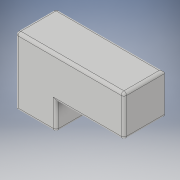
# Autodesk Inventor part: elbow
Saved by Autodesk Inventor 2019 (Build 230136000, 136)
## iProperties
Created: 2020-02-11
Part Number: elbow
Material: Generic
Document SubType Name: Modeling
Designer: Vinayak
Density: 1 g/cm^3
Appearance: Default
Author: Vinayak
Autodesk Inventor part; units mm, degrees
ref_plane "YZ Plane" through (0, 0, 0) normal (1, 0, 0) x (0, 1, 0)
ref_plane "XZ Plane" through (0, 0, 0) normal (0, 1, 0) x (-1, 0, 0)
ref_plane "XY Plane" through (0, 0, 0) normal (0, 0, 1) x (1, 0, 0)
sketch "Sketch1" plane through (0, 0, 0) normal (0, 0, 1) x (1, 0, 0)
  line L0 (0, 0) -> (-50, 0)
  line L1 (-50, 0) -> (-50, 30)
  line L2 (-50, 30) -> (0, 30)
  line L3 (0, 30) -> (0, 0)
  line L4 (-50, 30) -> (-80, 30)
  line L5 (-80, 30) -> (-80, -20)
  line L6 (-80, -20) -> (-50, -20)
  line L7 (-50, -20) -> (-50, 30)
  line L8 (-80, 0) -> (-50, 0)
  dimension "d0" = 50
  dimension "d1" = 30
  dimension "d2" = 30
  dimension "d3" = 50
  constraints: 18 end point, 4 parallel, 3 perpendicular, 2 horizontal, 1 point on line
  measures "d0" distance of L1.end L2.end
  measures "d1" distance of L0.end L1.end
  measures "d2" distance of L6.end L5.end
  measures "d3" distance of L5.end L4.end
extrude "Extrusion1" add sketch "Sketch1" along normal blind 30
fillet "Fillet1" radius 2 12 edges at (-40, 30, 30) (0, 15, 30) (-25, 0, 30) (-50, -10, 30) (-50, -20, 15) (-65, -20, 30) (0, 30, 15) (0, 0, 15) (-40, 30, 0) (-80, 30, 15) (-80, 5, 30) (-80, 5, 0)
body "Solid1"
